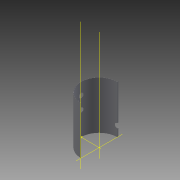
# Autodesk Inventor part: Upper Back Half 2014 Replacement
Saved by Autodesk Inventor 2015 (Build 190159000, 159)
## iProperties
Created: 2014-07-11
Part Number: Upper Back Half 2014 Replacement
Material: Generic
Document SubType Name: Modeling
Designer: I Rabey
Density: 1 g/cm^3
Appearance: Default
Author: I Rabey
Autodesk Inventor part; units mm, degrees
sketch "Sketch1" plane through (0, 0, 0) normal (0, 1, 0) x (-1, 0, 0)
  arc A0 (0, -307) -> (0, 307) centre (0, 0) ccw
  line L0 (0, 0) -> (0, 307) construction
  line L1 (0, 0) -> (0, -307) construction
  arc A1 (0, -308) -> (0, 308) centre (0, 0) ccw
  line L2 (0, 0) -> (0, 308) construction
  line L3 (0, 0) -> (0, -308) construction
  line L4 (0, 307) -> (0, 308)
  line L5 (0, -308) -> (0, -307)
  dimension "d0" = 307
  dimension "d1" = 180
  dimension "d2" = 308
  dimension "d3" = 180
  constraints: 12 end point, 4 point on circle, 2 centre point, 2 coincident, 1 collinear, 1 point on line
  measures "d0" radius of A0
  measures "d1" angle of L0 L1
  measures "d2" radius of A1
  measures "d3" angle of L2 L3
extrude "Extrusion1" add sketch "Sketch1" along normal blind 810.25
sketch "Sketch2" plane through (0, 0, 0) normal (0, 1, 0) x (-1, 0, 0)
  line L0 (0, 307) -> (1, 307)
  line L1 (1, 307) -> (1, 323)
  line L2 (1, 323) -> (0, 323)
  line L3 (0, 323) -> (0, 307)
  line L4 (0, -307) -> (1, -307)
  line L5 (1, -307) -> (1, -323)
  line L6 (1, -323) -> (0, -323)
  line L7 (0, -323) -> (0, -307)
  point P0 (0, 0)
  dimension "d6" = 1
  dimension "d7" = 16
  dimension "d8" = 1
  dimension "d9" = 16
  constraints: 16 end point, 4 parallel, 2 horizontal, 2 perpendicular
  measures "d6" distance of L2.end L1.end
  measures "d7" distance of L1.end L0.end
  measures "d8" distance of L5.end L6.end
  measures "d9" distance of L4.end L5.end
extrude "Extrusion2" add sketch "Sketch2" along normal blind 810.25
ref_plane "Work Plane1" through (-308, 0, 0) normal (-1, 0, 0) x (0, -1, 0)
sketch "Sketch3" plane through (-308, 0, 0) normal (-1, 0, 0) x (0, -1, 0)
  circle A0 centre (-395.75, 0) radius 38.5
  circle A1 centre (-610.75, 0) radius 38.5
  line L0 (0, -307.9984) -> (0, 307.9984) projected
  point P0 (0, 0)
  dimension "d15" = 77
  dimension "d16" = 77
  dimension "d20" = 395.75
  dimension "d21" = 610.75
  constraints: 2 centre point
  measures "d15" diameter of A0
  measures "d16" diameter of A1
  measures "d20" distance from line of L0 A0.centre
  measures "d21" distance from line of L0 A1.centre
extrude "Extrusion3" cut sketch "Sketch3" along normal blind 20 and the other way blind 20
ref_plane "Work Plane2" through (-1, 0, 307.9984) normal (-0.0032468, 0, 0.9999947) x (0.9999947, 0, 0.0032468)
ref_plane "Work Plane3" through (-1, 0, -307.9984) normal (-0.0032468, 0, -0.9999947) x (-0.9999947, 0, 0.0032468)
sketch "Sketch6" plane through (-1, 0, -307.9984) normal (-0.0032468, 0, -0.9999947) x (-0.9999947, 0, 0.0032468)
  line L0 (-0.9968, 0) -> (-0.9968, 810.25) projected
  circle A0 centre (-0.9968, 167.25) radius 38.5
  line L1 (0, 0) -> (308, 0) projected
  point P0 (2, 0)
  dimension "d40" = 77
  dimension "d41" = 167.25
  constraints: 1 centre point, 1 point on line
  measures "d40" diameter of A0
  measures "d41" distance from line of L1 A0.centre
extrude "Extrusion7" cut sketch "Sketch6" along normal blind 25 and the other way blind 25
body "Solid1"
